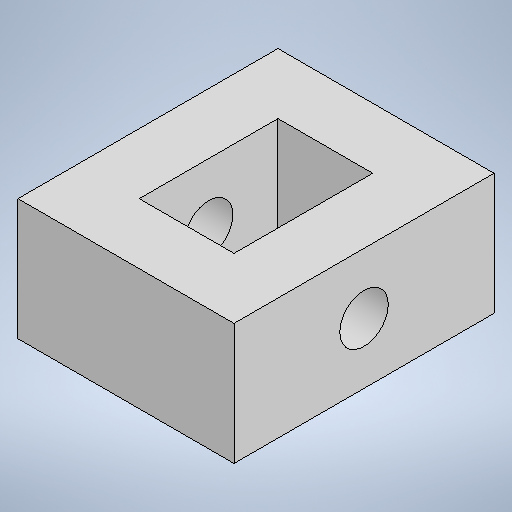
# Autodesk Inventor part: TopMotorMount
Saved by Autodesk Inventor 2026 (Build 300175050, 175E)
## iProperties
Created: 2025-12-26
Part Number: TopMotorMount
Material: Generic
Document SubType Name: Modeling
Designer: Nicholas M
Density: 1 g/cm^3
Appearance: Default
Author: Nicholas M
Autodesk Inventor part; units mm, degrees
ref_plane "YZ Plane" through (0, 0, 0) normal (1, 0, 0) x (0, 1, 0)
ref_plane "XZ Plane" through (0, 0, 0) normal (0, 1, 0) x (-1, 0, 0)
ref_plane "XY Plane" through (0, 0, 0) normal (0, 0, 1) x (1, 0, 0)
sketch "Sketch1" plane through (0, 0, 0) normal (0, 0, 1) x (1, 0, 0)
  line L0 (0, 0) -> (6.25, 0)
  line L1 (6.25, 0) -> (6.25, 8)
  line L2 (6.25, 8) -> (0, 8)
  line L3 (0, 8) -> (0, 0)
  line L4 (6.25, 0) -> (10.25, 0)
  line L5 (10.25, 0) -> (10.25, 8)
  line L6 (10.25, 8) -> (6.25, 8)
  line L7 (6.25, 8) -> (6.25, 0)
  line L8 (0, 0) -> (-4, 0)
  line L9 (-4, 0) -> (-4, 8)
  line L10 (-4, 8) -> (0, 8)
  line L11 (0, 8) -> (0, 0)
  point P0 (6.25, 4)
  point P1 (3.125, 8)
  dimension "d0" = 6.25
  dimension "d1" = 8
  dimension "d3" = 4
  constraints: 24 end point, 6 parallel, 3 horizontal, 3 perpendicular, 2 collinear, 2 midpoint, 1 point on line
  measures "d0" distance of L2.end L1.end
  measures "d1" distance of L0.end L1.end
  measures "d3" distance of L6.end L5.end
extrude "Extrusion1" add sketch "Sketch1" along normal blind 9.15 contours L8 L9 L10 L3 | L1 L6 L5 L4
extrude "Extrusion2" add sketch "Sketch1" against normal blind 4
sketch "Sketch2" plane through (10.25, 0, 9.15) normal (1, 0, 0) x (0, 0, -1)
  line L0 (9.15, 0) -> (9.15, 8) projected
  line L1 (9.15, 8) -> (0, 8) projected
  line L2 (0, 0) -> (0, 8) projected
  line L3 (9.15, 0) -> (0, 0) projected
  circle A0 centre (4.575, 4) radius 1.6
  line L4 (0, 0) -> (0, 8) projected
  point P0 (0, 4)
  point P1 (4.575, 8)
  dimension "d8" = 3.2
  constraints: 2 midpoint, 1 centre point, 1 horizontal alignment, 1 vertical alignment
  measures "d8" diameter of A0
extrude "Extrusion3" cut sketch "Sketch2" against normal through all contours A0
extrude "Extrusion4" add sketch "Sketch1" along normal blind 4 from surface at 9.15
body "Solid1"
